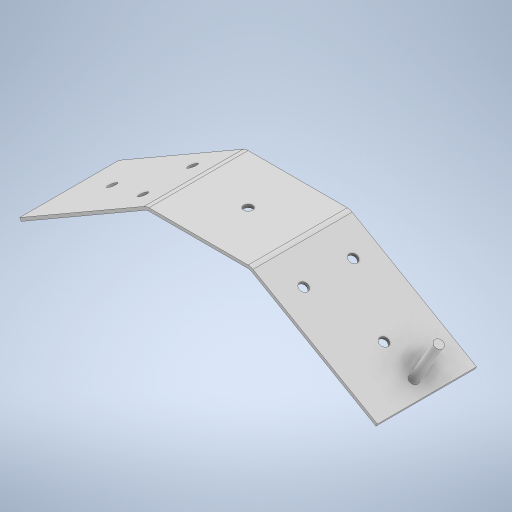
# Autodesk Inventor part: Obejma
Saved by Autodesk Inventor 2024 (Build 280153000, 153)
## iProperties
Created: 2024-11-18
Part Number: Obejma
Material: Generic
Document SubType Name: Modeling
Designer: Admin
Density: 1 g/cm^3
Appearance: Default
Mass: 196.464 g
Surface Area: 845.492 cm^2
Volume: 196.464 cm^3
Author: Admin
Autodesk Inventor part; units mm, degrees
ref_plane "YZ Plane" through (0, 0, 0) normal (1, 0, 0) x (0, 1, 0)
ref_plane "XZ Plane" through (0, 0, 0) normal (0, 1, 0) x (-1, 0, 0)
ref_plane "XY Plane" through (0, 0, 0) normal (0, 0, 1) x (1, 0, 0)
sketch "Sketch1" plane through (0, 0, 0) normal (0, 0, 1) x (1, 0, 0)
  line L0 (-200, 50) -> (200, 50)
  line L1 (200, 50) -> (200, -50)
  line L2 (200, -50) -> (-200, -50)
  line L3 (-200, -50) -> (-200, 50)
  line L4 (-200, 50) -> (200, -50) construction
  line L5 (200, 50) -> (-200, -50) construction
  point P0 (0, 0)
  dimension "d0" = 400
  dimension "d1" = 100
  constraints: 12 end point, 2 midpoint, 2 parallel, 1 horizontal, 1 perpendicular
  measures "d0" distance of L1.end L2.end
  measures "d1" distance of L0.end L1.end
extrude "Extrusion1" add sketch "Sketch1" along normal blind 3
sketch "Sketch2" plane through (0, 0, 3) normal (0, 0, 1) x (1, 0, 0)
  line L0 (200, 50) -> (-200, 50) projected
  line L1 (50, 50) -> (50, -50)
  line L2 (-200, -50) -> (200, -50) projected
  line L3 (-50, 50) -> (-50, -50)
  point P0 (0, 0)
  dimension "d4" = 100
  dimension "d5" = 50
  dimension "d6" = 50
  constraints: 4 end point, 3 point on line, 2 perpendicular
  measures "d4" distance of L1.start L1.end
  measures "d5" distance from line of point (0, 0) L1
  measures "d6" distance from line of point (0, 0) L3
bend part "Bend Part1" radius 10 angle 30 line through (-50, 50, 3) along (0, -1, 0) centre toward (0, 0, -1) moving side (-1, 0, 0) both sides no
sketch "Sketch3" plane through (0, 0, 3) normal (0, 0, 1) x (1, 0, 0)
  line L0 (50, 50.2356) -> (50, -50)
  line L1 (-50, -50) -> (200, -50) projected
  point P0 (0, 0)
  dimension "d9" = 50
  constraints: 2 end point, 1 point on line, 1 vertical
  measures "d9" distance from line of point (0, 0) L0
bend part "Bend Part2" radius 10 angle 30 line through (50, 50.2356, 3) along (0, -1, 0) centre toward (0, 0, -1) moving side (1, 0, 0) both sides no
sketch "Sketch4" plane through (0, 0, 3) normal (0, 0, 1) x (1, 0, 0)
  circle A0 centre (0, 0) radius 4.5
  dimension "d12" = 9
  constraints: 1 centre point, 1 coincident
  measures "d12" diameter of A0
extrude "Extrusion2" cut sketch "Sketch4" against normal blind 5
sketch "Sketch5" plane through (55, -50, 1.6603) normal (0.5, 0, 0.8660254) x (0.8660254, 0, -0.5)
  circle A0 centre (30, 25) radius 4.5
  circle A1 centre (30, 75) radius 4.5
  line L0 (0, 0) -> (144.764, 0) projected
  line L1 (0, 100) -> (0, 0) projected
  circle A2 centre (94.764, 50) radius 4.5
  line L2 (144.764, 0) -> (144.764, 100) projected
  line L3 (144.764, 100) -> (0, 100) projected
  circle A3 centre (129.764, 50) radius 4.5
  point P0 (-46.8013, 50)
  dimension "d15" = 9
  dimension "d16" = 9
  dimension "d17" = 50
  dimension "d18" = 25
  dimension "d19" = 30
  dimension "d20" = 30
  dimension "d31" = 9
  dimension "d32" = 50
  dimension "d33" = 50
  dimension "d37" = 9
  dimension "d38" = 50
  dimension "d44" = 35
  constraints: 4 centre point
  measures "d15" diameter of A0
  measures "d16" diameter of A1
  measures "d17" distance of A1.centre A0.centre
  measures "d18" distance from line of L0 A0.centre
  measures "d19" distance from line of L1 A0.centre
  measures "d20" distance from line of L1 A1.centre
  measures "d31" diameter of A2
  measures "d32" distance from line of L2 A2.centre
  measures "d33" distance from line of L3 A2.centre
  measures "d37" diameter of A3
  measures "d38" distance from line of L0 A3.centre
  measures "d44" distance of A2.centre A3.centre
extrude "Extrusion3" cut sketch "Sketch5" against normal blind 5 contours A0 | A1 | A2
sketch "Sketch6" plane through (-55, -50, 1.6603) normal (-0.5, 0, 0.8660254) x (0.8660254, 0, 0.5)
  circle A0 centre (-30, 75) radius 4.5
  circle A1 centre (-30, 25) radius 4.5
  line L0 (0, 100) -> (-144.764, 100) projected
  line L1 (0, 0) -> (0, 100) projected
  circle A2 centre (-94.764, 50) radius 4.5
  line L2 (-144.764, 100) -> (-144.764, 0) projected
  point P0 (46.8013, 50)
  dimension "d23" = 9
  dimension "d24" = 9
  dimension "d25" = 25
  dimension "d26" = 50
  dimension "d27" = 30
  dimension "d28" = 30
  dimension "d34" = 9
  dimension "d35" = 50
  dimension "d36" = 50
  constraints: 3 centre point
  measures "d23" diameter of A0
  measures "d24" diameter of A1
  measures "d25" distance from line of L0 A0.centre
  measures "d26" distance of A0.centre A1.centre
  measures "d27" distance from line of L1 A0.centre
  measures "d28" distance from line of L1 A1.centre
  measures "d34" diameter of A2
  measures "d35" distance from line of L2 A2.centre
  measures "d36" distance from line of L0 A2.centre
extrude "Extrusion4" cut sketch "Sketch6" against normal blind 5
sketch "Sketch7" plane through (55, -50, 1.6603) normal (0.5, 0, 0.8660254) x (0.8660254, 0, -0.5)
  circle A0 centre (129.764, 50) radius 4.5
  line L0 (144.764, 0) -> (144.764, 100) projected
  line L1 (0, 0) -> (144.764, 0) projected
  point P0 (-46.8013, 50)
  dimension "d45" = 9
  dimension "d46" = 15
  dimension "d47" = 50
  constraints: 1 centre point
  measures "d45" diameter of A0
  measures "d46" distance from line of L0 A0.centre
  measures "d47" distance from line of L1 A0.centre
extrude "Extrusion5" add sketch "Sketch7" along normal blind 50
body "Solid1"
